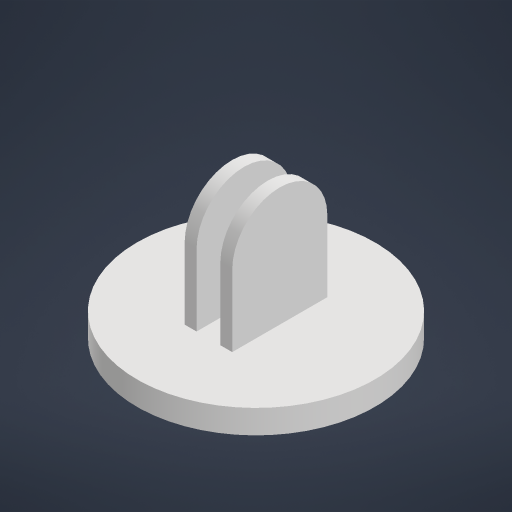
# Autodesk Inventor part: Base-Arm Connector
Saved by Autodesk Inventor 2023.1 (Build 271208000, 208)
## iProperties
Created: 2022-12-06
Part Number: Base-Arm Connector
Material: Generic
Document SubType Name: Modeling
Designer: aubrey-work
Density: 1 g/cm^3
Appearance: Default
Author: aubrey-work
Autodesk Inventor part; units mm, degrees
ref_plane "YZ Plane" through (0, 0, 0) normal (1, 0, 0) x (0, 1, 0)
ref_plane "XZ Plane" through (0, 0, 0) normal (0, 1, 0) x (-1, 0, 0)
ref_plane "XY Plane" through (0, 0, 0) normal (0, 0, 1) x (1, 0, 0)
sketch "Sketch1" plane through (0, 0, 0) normal (0, 1, 0) x (-1, 0, 0)
  circle A0 centre (0, 0) radius 127
  dimension "swivelBaseDiameter" = 254
  constraints: 1 centre point, 1 coincident
  measures "swivelBaseDiameter" diameter of A0
extrude "Extrusion1" add sketch "Sketch1" along normal blind 25.4
sketch "Sketch2" plane through (0, 25.4, 0) normal (0, 1, 0) x (1, 0, 0)
  circle A0 centre (0, 0) radius 127 construction
  line L0 (0, -127) -> (0, 127) construction
  line L1 (-25.4, 50.8) -> (-12.7, 50.8)
  line L2 (-12.7, 50.8) -> (-12.7, -50.8)
  line L3 (-12.7, -50.8) -> (-25.4, -50.8)
  line L4 (-25.4, -50.8) -> (-25.4, 50.8)
  line L5 (-127, 0) -> (127, 0) construction
  line L6 (25.4, 50.8) -> (12.7, 50.8)
  line L7 (12.7, 50.8) -> (12.7, -50.8)
  line L8 (12.7, -50.8) -> (25.4, -50.8)
  line L9 (25.4, -50.8) -> (25.4, 50.8)
  point P0 (-12.7, 0)
  point P1 (12.7, 0)
  dimension "armConnectorSeparation" = 12.7
  dimension "armConnectorsThickness" = 12.7
  dimension "armConnectorsSize" = 101.6
  constraints: 20 end point, 5 symmetric about line, 4 point on circle, 3 midpoint, 2 horizontal, 2 parallel, 1 perpendicular, 1 point on line, 1 vertical
  measures "armConnectorSeparation" distance between parallel lines of L2 L0
  measures "armConnectorsThickness" distance of L1.start L1.end
  measures "armConnectorsSize" distance of L1.end L2.end
extrude "Extrusion2" add sketch "Sketch2" along normal blind 25.4
sketch "Sketch3" plane through (25.4, 25.4, 50.8) normal (1, 0, 0) x (0, 0, -1)
  circle A0 centre (50.8, 76.2) radius 50.8 construction
  line L0 (101.6, 25.4) -> (101.6, 76.2)
  line L1 (0, 25.4) -> (0, 76.2)
  arc A1 (101.6, 76.2) -> (0, 76.2) centre (50.8, 76.2) ccw
  line L2 (0, 25.4) -> (101.6, 25.4)
  point P0 (50.8, 25.4)
  dimension "d9" = 101.6
  constraints: 6 end point, 5 point on circle, 3 tangent, 2 centre point, 2 point on line, 1 midpoint, 1 parallel, 1 perpendicular, 1 vertical
  measures "d9" diameter of A0
extrude "Extrusion3" add sketch "Sketch3" against normal up to surface (12.7 mm away)
extrude "Extrusion4" add sketch "Sketch3" against normal up to surface (12.7 mm away) from surface at -38.1
equation "\"d9\" = armConnectorsSize"
equation "\"d10\" = armConnectorsSize"
body "Solid1"
